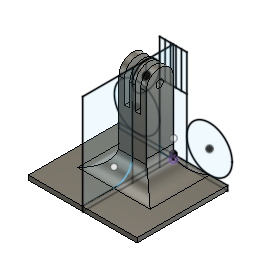
phone_holder_base (Autodesk Fusion 360 design; units mm, degrees)
Autodesk Fusion 360 part; units mm, degrees
note: some values were not read from the file. Set by a fixed rule: which sketch regions a step uses.
sketch "Sketch1" plane through (0, 0, 0) normal (0, 0, 1) x (1, 0, 0)
  line L0 (-38.1, 0) -> (38.1, 0)
  line L1 (-9.525, 0) -> (9.525, 0)
  line L2 (9.525, 0) -> (9.525, 69.85)
  line L3 (9.525, 69.85) -> (-9.525, 69.85)
  line L4 (-9.525, 69.85) -> (-9.525, 0)
  line L5 (-38.1, 0) -> (-38.1, 3.175)
  line L6 (-38.1, 3.175) -> (38.1, 3.175)
  line L7 (38.1, 3.175) -> (38.1, 0)
  circle A0 centre (-25.4, 19.05) radius 15.875
  circle A1 centre (25.4, 19.05) radius 15.875
  line L8 (-9.525, 44.45) -> (9.525, 44.45)
  line L9 (-5.715, 69.85) -> (-5.715, 44.45)
  line L10 (-1.905, 69.85) -> (-1.905, 44.45)
  line L11 (1.905, 69.85) -> (1.905, 44.45)
  line L12 (5.715, 69.85) -> (5.715, 44.45)
  dimension "d2" = 19.05
  dimension "d3" = 9.525
  dimension "d4" = 3.175
  dimension "d5" = 76.2
  dimension "d6" = 31.75
  dimension "d7" = 31.75
  dimension "d17" = 69.85
  dimension "d18" = 3.175
  dimension "d28" = 25.4
  dimension "d29" = 3.81
  dimension "d30" = 3.81
  dimension "d31" = 3.81
  dimension "d32" = 3.81
  constraint horizontal L0
  constraint midpoint origin L0
  constraint horizontal L1
  constraint vertical L2
  constraint horizontal L3
  constraint vertical L4
  constraint coincident L0 L1.start
  constraint perpendicular L0 L5
  constraint perpendicular L5 L6
  constraint tangent L4 A0
  constraint tangent L6 A0
  constraint tangent L2 A1
  constraint tangent L6 A1
  constraint coincident L4 L8.start
  constraint coincident L2 L8.end
  constraint perpendicular L2 L8
  constraint coincident L3 L9.start
  constraint coincident L8 L9.end
  constraint perpendicular L8 L9
  constraint coincident L3 L10.start
  constraint coincident L8 L10.end
  constraint perpendicular L8 L10
  constraint coincident L3 L11.start
  constraint coincident L8 L11.end
  constraint perpendicular L8 L11
  constraint coincident L3 L12.start
  constraint coincident L8 L12.end
  constraint perpendicular L8 L12
  measures "d2" distance of L2.end L3.end
  measures "d3" distance of origin L4
  measures "d4" distance of L0.start L5.end
  measures "d5" distance of L5.end L6.end
  measures "d6" diameter of A0
  measures "d7" diameter of A1
  measures "d17" distance of L0 L3
  measures "d18" distance of L0.end L6.end
  measures "d28" distance of L3 L8
  measures "d29" distance of L3.end L9.start
  measures "d30" distance of L9 L10
  measures "d31" distance of L10 L11.start
  measures "d32" distance of L11 L12
extrude "Extrude1" add sketch "Sketch1" along normal blind 63.5 contours L0 L4 L5 L6 | L0 L1 L2 L4 L6 | L0 L2 L6 L7 | L4 L6 A0 | L2 L4 L6 L8 | L2 L6 A1 | L3 L4 L8 L9 | L2 L3 L8 L12 | L3 L8 L9 L10 | L3 L8 L11 L12 | L3 L8 L10 L11 makes body 1
sketch "Sketch3" plane through (0, 0, 0) normal (1, 0, 0) x (0, 0, -1)
  line L0 (0, 0) -> (-63.5, 0)
  line L1 (-63.5, 0) -> (-63.5, 69.85)
  line L2 (-63.5, 69.85) -> (0, 69.85)
  line L3 (0, 69.85) -> (0, 0)
  line L4 (-63.5, 3.175) -> (0, 3.175)
  line L5 (-19.05, 69.85) -> (-19.05, 0)
  line L6 (0, 3.175) -> (0, 0)
  line L7 (-9.525, 69.85) -> (-9.525, 0)
  line L8 (-28.575, 69.85) -> (-28.575, 0)
  circle A0 centre (-19.05, 60.325) radius 9.525
  arc A1 (-9.525, 13.9553) -> (0, 3.175) centre (0, 12.7731) ccw
  arc A2 (-41.5769, 3.175) -> (-28.575, 16.6144) centre (-41.5769, 16.184) ccw
  circle A3 centre (-19.05, 60.325) radius 2.54
  circle A4 centre (-19.05, 60.325) radius 2.032
  dimension "d15" = 63.5
  dimension "d16" = 69.85
  dimension "d19" = 3.175
  dimension "d20" = 19.05
  dimension "d21" = 9.525
  dimension "d22" = 9.525
  dimension "d23" = 19.05
  dimension "d25" = 5.08
  dimension "d35" = 4.064
  constraint horizontal L0
  constraint vertical L1
  constraint horizontal L2
  constraint vertical L3
  constraint coincident L0.start L3.end
  constraint coincident L1 L4.start
  constraint coincident L3 L4.end
  constraint perpendicular L3 L4
  constraint coincident L2 L5.start
  constraint coincident L0 L5.end
  constraint perpendicular L0 L5
  constraint coincident L2 L7.start
  constraint coincident L0 L7.end
  constraint perpendicular L0 L7
  constraint coincident L2 L8.start
  constraint coincident L0 L8.end
  constraint perpendicular L0 L8
  constraint coincident L5 A0.centre
  constraint coincident L5.start A0
  constraint tangent L4 A1
  constraint coincident L4.end L6.start
  constraint coincident L7 A1.start
  constraint tangent L4 A2
  constraint coincident L4 A2.start
  constraint coincident L8 A2.end
  constraint concentric A0 A3
  constraint concentric A3 A4
  measures "d15" distance of L0.start L0.end
  measures "d16" distance of L0.start L2.end
  measures "d19" distance of L0.end L4
  measures "d20" distance of L5 L6
  measures "d21" distance of L5.start L7.start
  measures "d22" distance of L5.start L8.start
  measures "d23" diameter of A0
  measures "d25" diameter of A3
  measures "d35" diameter of A4
extrude "Extrude2" cut sketch "Sketch3" along normal mid plane 81.28 contours L2 L3 L7 A1 | L2 L7 A0 | L2 L8 A0 | L1 L2 L4 L8 A2 | L5 A3 A4 | L5 A3 A4 | L5 A4 | L5 A4 bodies 1
extrude "Extrude3" cut sketch "Sketch1" along normal blind 33.02 contours L3 L8 L9 L10 | L3 L8 L11 L12 bodies 1
extrude "Extrude4" add sketch "Sketch3" along normal blind -9.525 and the other way blind 5.715 contours L5 A3 A4 | L5 A3 A4 bodies 1
copy_body "Body->Comp1" bodies 1 removing the originals makes body 2 in component "Base"
component "Base" placed x (1, 0, 0) y (0, 1, 0) z (0, 0, 1) at (0, 0, 0)
